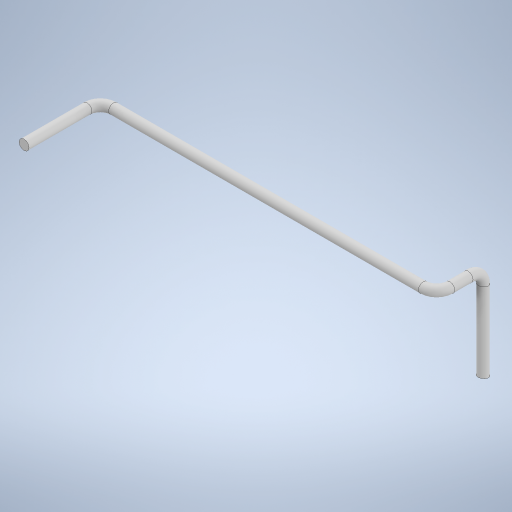
# Autodesk Inventor part: HUDSON-1-86
Saved by Autodesk Inventor 2024.2 (Build 282272000, 272)
## iProperties
Created: 2024-10-10
Part Number: HUDSON-1-86
Material: Generic
Document SubType Name: Modeling
Designer: Precisión-10
Density: 1 g/cm^3
Appearance: Default
Author: Precisión-10
Autodesk Inventor part; units mm, degrees
ref_plane "YZ Plane" through (0, 0, 0) normal (1, 0, 0) x (0, 1, 0)
ref_plane "XZ Plane" through (0, 0, 0) normal (0, 1, 0) x (-1, 0, 0)
sketch "Sketch2" plane through (0, 0, 0) normal (0, 1, 0) x (-1, 0, 0)
  line L0 (0, 0) -> (0, 5.5)
  line L1 (4, 9.5) -> (97.5, 9.5)
  arc A0 (4, 9.5) -> (0, 5.5) centre (4, 5.5) ccw
  arc A1 (97.5, 9.5) -> (101.5, 13.5) centre (97.5, 13.5) ccw
  line L2 (101.5, 13.5) -> (101.5, 32.5)
  point P0 (0, 9.5)
  dimension "d2" = 97.5
  dimension "d3" = 4
  dimension "d12" = 8
  dimension "d13" = 19
  dimension "d14" = 5.5
  constraints: 6 end point, 4 point on circle, 4 tangent, 2 centre point, 2 point on line, 2 vertical, 1 perpendicular
  measures "d2" distance of point (0, 9.5) L1.end
  measures "d3" radius of A0
  measures "d12" diameter of A1
  measures "d13" distance of L2.start L2.end
  measures "d14" distance of L0.start L0.end
sketch "Sketch1" plane through (0, 0, 0) normal (0, 0, 1) x (1, 0, 0)
  circle A0 centre (0, 0) radius 1.5
  dimension "d0" = 3
  constraints: 1 centre point, 1 coincident
  measures "d0" diameter of A0
sweep "Sweep1" add profiles "Sketch1" path "Sketch2"
ref_plane "Work Plane4" through (-97.5, 0, 9.5) normal (-1, 0, 0) x (0, -1, 0)
sketch "Sketch6" plane through (0, 0, 0) normal (1, 0, 0) x (0, 1, 0)
  line L0 (1.5, 0) -> (-1.5, 0) construction
  line L1 (-27.9686, -4.5003) -> (-3.9686, -4.5003)
  arc A0 (-3.9686, -4.5003) -> (0, 0) centre (-3.9686, -0.5003) ccw
  line L2 (1.5, 5.5) -> (-1.5, 5.5) projected
  line L3 (1.5, 0) -> (-1.5, 0) projected
  line L4 (1.5, 0) -> (-1.5, 0) projected
  point P0 (-6.0857, 0)
  dimension "d19" = 24
  dimension "d20" = 4
  constraints: 5 point on circle, 4 midpoint, 2 end point, 1 centre point, 1 tangent
  measures "d19" distance of L1.start L1.end
  measures "d20" radius of A0
sketch "Sketch7" plane through (0, 0, 0) normal (0, 0, -1) x (-1, 0, 0)
  circle A0 centre (0, 0) radius 1.5
  dimension "d21" = 3
  constraints: 1 centre point, 1 coincident
  measures "d21" diameter of A0
sweep "Sweep2" add profiles "Sketch7" path "Sketch6" path curves A0 L1
body "Solid1"
